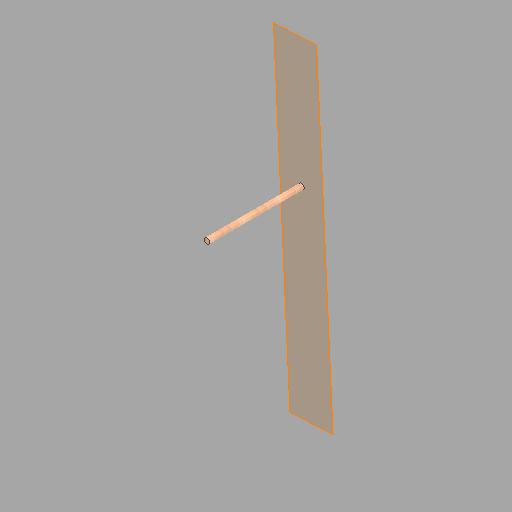
# Autodesk Inventor part: PIPE
Saved by Autodesk Inventor 2025.2 (Build 292293000, 293)
## iProperties
Created: 2025-01-27
Part Number: PIPE
Material: Wood (Birch)
Document SubType Name: Modeling
Designer: Anna
Density: 0.55 g/cm^3
Appearance: Birch - Natural Polished
Mass: 422.068 g
Surface Area: 828.467 cm^2
Volume: 767.396 cm^3
Author: Anna
Autodesk Inventor part; units mm, degrees
ref_plane "Work Plane1" through (13.18, 611.2067, 0) normal (0, 0, 1) x (0.9987, 0.05, 0)
sketch "Sketch1" plane through (13.18, 611.2067, 0) normal (0, 0, 1) x (0.9987, 0.05, 0)
  circle A0 centre (0, 255) radius 19.05
  point P0 (-43.7171, -609.7837)
  dimension "d0" = 38.1
  constraints: 1 centre point
  measures "d0" diameter of A0
ref_plane "Work Plane2" through (-139.7, -1066.8, 927.1) normal (0, 0, -1) x (0, 1, 0)
ref_plane "Work Plane3" through (-1119.7006, 442.527, 939.8) normal (0, 0, -1) x (0.2879, 0.9577, 0)
ref_plane "Work Plane4" through (-1119.7006, 442.527, 673.1) normal (0, 0, -1) x (0.2879, 0.9577, 0)
extrude "Extrusion1" add sketch "Sketch1" along normal up to surface (673.1 mm away)
body "Solid1"
